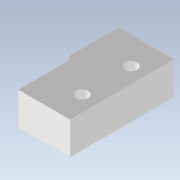
# Autodesk Inventor part: MicroswitchBig
Saved by Autodesk Inventor 2022.1 (Build 261234020, 234B)
## iProperties
Created: 2022-07-13
Part Number: MicroswitchBig
Material: Generisch
Document SubType Name: Modeling
Designer: Rama
Density: 1 g/cm^3
Appearance: Vorgabe
Author: Rama
Autodesk Inventor part; units mm, degrees
ref_plane "YZ Plane" through (0, 0, 0) normal (1, 0, 0) x (0, 1, 0)
ref_plane "XZ Plane" through (0, 0, 0) normal (0, 1, 0) x (-1, 0, 0)
ref_plane "XY Plane" through (0, 0, 0) normal (0, 0, 1) x (1, 0, 0)
sketch "Skizze1" plane through (0, 0, 0) normal (0, 1, 0) x (-1, 0, 0)
  line L0 (-5.35, 10.05) -> (5.35, 10.05)
  line L1 (5.35, 10.05) -> (5.35, -10.05)
  line L2 (5.35, -10.05) -> (-5.35, -10.05)
  line L3 (-5.35, -10.05) -> (-5.35, 10.05)
  line L4 (-5.35, 10.05) -> (5.35, -10.05) construction
  line L5 (5.35, 10.05) -> (-5.35, -10.05) construction
  line L6 (4.61, 10.05) -> (4.61, 0.15)
  line L7 (4.61, 0.15) -> (5.35, -0.59)
  point P0 (0, 0)
  dimension "d0" = 10.7
  dimension "d1" = 20.1
  dimension "d2" = 9.96
  dimension "d3" = 9.9
  dimension "d4" = 45
  constraints: 16 end point, 2 midpoint, 2 parallel, 2 point on line, 1 horizontal, 1 perpendicular, 1 vertical
  measures "d0" distance of L1.end L2.end
  measures "d1" distance of L0.end L1.end
  measures "d2" distance between parallel lines of L3 L6
  measures "d3" distance from line of L0 L6.end
  measures "d4" angle of L1 L7
extrude "Extrusion1" add sketch "Skizze1" along normal blind 6.35 contours L0 L6 L7 L1 L2 L3
sketch "Skizze2" plane through (-5.35, 0, -10.05) normal (-1, 0, 0) x (0, 0, 1)
  line L0 (6, 4.5) -> (8.03, 4.5)
  line L1 (8.03, 4.5) -> (8.03, 1.05)
  line L2 (8.03, 1.05) -> (6, 1.05)
  line L3 (6, 1.05) -> (6, 4.5)
  line L4 (0, 0) -> (9.46, 0) projected
  line L5 (0, 6.35) -> (9.46, 6.35) projected
  line L6 (0, 0) -> (0, 6.35) projected
  point P0 (10.05, 0)
  dimension "d7" = 2.03
  dimension "d8" = 3.45
  dimension "d9" = 1.05
  dimension "d10" = 1.85
  dimension "d11" = 6
  constraints: 8 end point, 2 parallel, 1 horizontal, 1 perpendicular
  measures "d7" distance of L1.end L2.end
  measures "d8" distance of L0.end L1.end
  measures "d9" distance between parallel lines of L4 L2
  measures "d10" distance between parallel lines of L5 L0
  measures "d11" distance between parallel lines of L6 L3
extrude "Extrusion2" add sketch "Skizze2" along normal blind 1.6
fillet "Rundung1" radius 0.8 2 edges at (-6.95, 2.775, -2.02) (-6.95, 2.775, -4.05)
sketch "Skizze3" plane through (0, 6.35, 0) normal (0, 1, 0) x (1, 0, 0)
  line L0 (-4.61, -0.15) -> (-4.61, -10.05) projected
  line L1 (5.35, -10.05) -> (5.35, 10.05) projected
  line L2 (5.35, 10.05) -> (-5.35, 10.05) projected
  line L3 (-4.61, -10.05) -> (5.35, -10.05) projected
  point P0 (0, 0)
  point P1 (2.31, -4.75)
  point P2 (2.31, 4.75)
  dimension "d15" = 9.5
  dimension "d16" = 6.92
  dimension "d17" = 3.04
  dimension "d18" = 0
  dimension "d19" = 5.3
  dimension "d20" = 5.3
  measures "d15" distance of point (2.31, 4.75) point (2.31, -4.75)
  measures "d16" distance from line of point (2.31, -4.75) L0
  measures "d17" distance from line of point (2.31, -4.75) L1
  measures "d18" horizontal distance of point (2.31, -4.75) point (2.31, 4.75)
  measures "d19" distance from line of point (2.31, 4.75) L2
  measures "d20" distance from line of point (2.31, -4.75) L3
hole "Bohrung1" at (2.31, 6.35, 4.75) at (2.31, 6.35, -4.75) direction (0, -1, 0) diameter 2.5 end through all
sketch "Skizze4" plane through (-6.95, 0, -10.05) normal (-1, 0, 0) x (0, 0, 1)
  line L0 (6.8, 1.05) -> (6.8, 4.5) projected
  line L1 (6.8, 1.05) -> (7.23, 1.05) projected
  line L2 (7.23, 4.5) -> (7.23, 1.05) projected
  line L3 (7.23, 4.5) -> (6.8, 4.5) projected
  circle A0 centre (7.015, 2.775) radius 0.1
  point P0 (10.05, 0)
  dimension "d28" = 0.2
  dimension "d29" = 1.725
  dimension "d30" = 1.725
  dimension "d31" = 0.43
  dimension "d32" = 0.215
  constraints: 1 centre point
  measures "d28" diameter of A0
  measures "d29" distance from line of A0.centre L3
  measures "d30" distance from line of A0.centre L1
  measures "d31" distance between parallel lines of L2 L0
  measures "d32" distance from line of A0.centre L0
extrude "Extrusion3" cut sketch "Skizze4" against normal blind 0.2 contours A0
equation "\"d19\" = d20"
equation "\"d32\" = 0.5 * d31"
